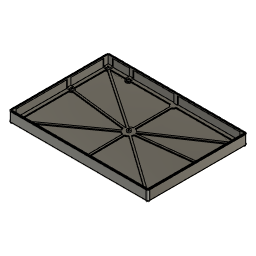
bottom (Autodesk Fusion 360 design; units mm, degrees)
Autodesk Fusion 360 part; units mm, degrees
note: some values were not read from the file. Set by a fixed rule: which sketch regions a step uses.
sketch "Szkic1" plane through (0, 0, 0) normal (0, 0, 1) x (1, 0, 0)
  line L0 (-4, -4) -> (301, -4)
  line L1 (301, -4) -> (301, 214)
  line L2 (301, 214) -> (-4, 214)
  line L3 (-4, 214) -> (-4, -4)
  circle A0 centre (5, 205) radius 1.6
  circle A1 centre (50, 205) radius 1.6
  circle A2 centre (292, 205) radius 1.6
  circle A3 centre (292, 5) radius 1.6
  circle A4 centre (148.5, 5) radius 1.6
  circle A5 centre (5, 5) radius 1.6
  circle A6 centre (147.5, 108) radius 1.6
  circle A7 centre (5, 125) radius 1.6
  circle A8 centre (292, 125) radius 1.6
  dimension "d1" = 4
  dimension "d2" = 4
  dimension "d3" = 214
  dimension "d4" = 301
  dimension "d5" = 3.2
  dimension "d6" = 3.2
  dimension "d7" = 3.2
  dimension "d8" = 3.2
  dimension "d9" = 3.2
  dimension "d10" = 3.2
  dimension "d11" = 3.2
  dimension "d12" = 3.2
  dimension "d13" = 3.2
  dimension "d14" = 205
  dimension "d15" = 5
  dimension "d16" = 50
  dimension "d17" = 292
  dimension "d18" = 5
  dimension "d19" = 5
  dimension "d20" = 148.5
  dimension "d22" = 292
  dimension "d24" = 125
  dimension "d25" = 108
  dimension "d26" = 147.5
  constraint horizontal L0
  constraint vertical L1
  constraint horizontal L2
  constraint vertical L3
  constraint horizontal A0.centre A1.centre
  constraint horizontal A1.centre A2.centre
  constraint horizontal A4.centre A5.centre
  constraint horizontal A3.centre A4.centre
  constraint horizontal A7.centre A8.centre
  constraint vertical A3.centre A8.centre
  constraint vertical A5.centre A7.centre
  measures "d1" horizontal distance of origin L0.start
  measures "d2" vertical distance of origin L0.start
  measures "d3" vertical distance of origin L2.end
  measures "d4" horizontal distance of origin L0.end
  measures "d5" diameter of A0
  measures "d6" diameter of A1
  measures "d7" diameter of A7
  measures "d8" diameter of A6
  measures "d9" diameter of A8
  measures "d10" diameter of A2
  measures "d11" diameter of A5
  measures "d12" diameter of A4
  measures "d13" diameter of A3
  measures "d14" vertical distance of origin A0.centre
  measures "d15" horizontal distance of origin A0.centre
  measures "d16" horizontal distance of origin A1.centre
  measures "d17" horizontal distance of origin A2.centre
  measures "d18" horizontal distance of origin A5.centre
  measures "d19" vertical distance of origin A5.centre
  measures "d20" horizontal distance of origin A4.centre
  measures "d22" horizontal distance of origin A8.centre
  measures "d24" vertical distance of origin A7.centre
  measures "d25" vertical distance of origin A6.centre
  measures "d26" horizontal distance of origin A6.centre
extrude "Wyciągnięcie proste1" add sketch "Szkic1" along normal blind 4
sketch "Szkic2" plane through (0, 0, 0) normal (0, 0, -1) x (1, 0, 0)
  circle A0 centre (292, -205) radius 1.6
  circle A1 centre (5, -205) radius 1.6
  circle A2 centre (50, -205) radius 1.6
  circle A3 centre (292, -5) radius 1.6
  circle A4 centre (148.5, -5) radius 1.6
  circle A5 centre (5, -5) radius 1.6
  circle A6 centre (147.5, -108) radius 1.6
  circle A7 centre (5, -125) radius 1.6
  circle A8 centre (292, -125) radius 1.6
  line L0 (-4, 4) -> (-4, -214)
  line L1 (-4, -214) -> (301, -214)
  line L2 (301, -214) -> (301, 4)
  line L3 (301, 4) -> (-4, 4)
  circle A9 centre (5, -5) radius 3
  circle A10 centre (148.5, -5) radius 3
  circle A11 centre (292, -5) radius 3
  circle A12 centre (292, -125) radius 3
  circle A13 centre (147.5, -108) radius 3
  circle A14 centre (5, -125) radius 3
  circle A15 centre (5, -205) radius 3
  circle A16 centre (50, -205) radius 3
  circle A17 centre (292, -205) radius 3
  dimension "d29" = 6
  dimension "d30" = 6
  dimension "d31" = 6
  dimension "d32" = 6
  dimension "d33" = 6
  dimension "d34" = 6
  dimension "d35" = 6
  dimension "d36" = 6
  dimension "d37" = 6
  constraint concentric A5 A9
  constraint concentric A4 A10
  constraint concentric A3 A11
  constraint concentric A8 A12
  constraint concentric A6 A13
  constraint concentric A7 A14
  constraint concentric A1 A15
  constraint concentric A2 A16
  constraint concentric A0 A17
  measures "d29" diameter of A9
  measures "d30" diameter of A10
  measures "d31" diameter of A11
  measures "d32" diameter of A12
  measures "d33" diameter of A13
  measures "d34" diameter of A14
  measures "d35" diameter of A15
  measures "d36" diameter of A16
  measures "d37" diameter of A17
extrude "Wyciągnięcie proste2" cut sketch "Szkic2" against normal blind 2 contours A9 | A10 | A11 | A12 | A13 | A14 | A15 | A16 | A17
sketch "Szkic3" plane through (0, 0, 4) normal (0, 0, 1) x (-1, 0, 0)
  circle A0 centre (-292, -205) radius 1.6
  circle A1 centre (-5, -205) radius 1.6
  circle A2 centre (-50, -205) radius 1.6
  circle A3 centre (-292, -5) radius 1.6
  circle A4 centre (-148.5, -5) radius 1.6
  circle A5 centre (-5, -5) radius 1.6
  circle A6 centre (-147.5, -108) radius 1.6
  circle A7 centre (-5, -125) radius 1.6
  circle A8 centre (-292, -125) radius 1.6
  line L0 (4, -214) -> (4, 4)
  line L1 (4, 4) -> (-301, 4)
  line L2 (-301, 4) -> (-301, -214)
  line L3 (-301, -214) -> (4, -214)
  circle A9 centre (-5, -205) radius 6
  circle A10 centre (-50, -205) radius 6
  circle A11 centre (-147.5, -108) radius 12
  circle A12 centre (-5, -125) radius 6
  circle A13 centre (-5, -5) radius 6
  circle A14 centre (-292, -205) radius 6
  circle A15 centre (-292, -125) radius 6
  circle A16 centre (-148.5, -5) radius 6
  circle A17 centre (-292, -5) radius 6
  line L4 (-5, -205) -> (-147.5, -108)
  line L5 (-147.5, -108) -> (-5, -125)
  line L6 (-5, -125) -> (-5, -205)
  line L7 (-5, -5) -> (-5, -125)
  line L8 (-5, -5) -> (-147.5, -108)
  line L9 (-147.5, -108) -> (-148.5, -5)
  line L10 (-148.5, -5) -> (-5, -5)
  line L11 (-148.5, -5) -> (-292, -5)
  line L12 (-292, -5) -> (-147.5, -108)
  line L13 (-147.5, -108) -> (-292, -125)
  line L14 (-292, -125) -> (-292, -5)
  line L15 (-292, -125) -> (-292, -205)
  line L16 (-292, -205) -> (-147.5, -108)
  line L17 (-5, -205) -> (-50, -205)
  line L18 (-50, -205) -> (-292, -205)
  circle A18 centre (-147.5, -205) radius 6
  line L19 (-147.5, -108) -> (-147.5, -205)
  line L20 (-10.8017, -203.4702) -> (-138.8443, -116.3113)
  line L21 (-145.5, -119.8322) -> (-145.5, -199.3431)
  line L22 (-149.5, -119.8322) -> (-149.5, -199.3431)
  line L23 (-286.1885, -203.5077) -> (-156.2093, -116.2552)
  line L24 (-288.4179, -200.1866) -> (-158.4387, -112.9341)
  line L25 (-159.0174, -111.3688) -> (-286.1482, -126.3253)
  line L26 (-286.6156, -122.3527) -> (-159.4848, -107.3962)
  line L27 (-158.2959, -102.7608) -> (-288.5545, -9.9121)
  line L28 (-286.2327, -6.6548) -> (-155.9741, -99.5036)
  line L29 (-149.6148, -96.1878) -> (-150.445, -10.676)
  line L30 (-146.4452, -10.6372) -> (-145.615, -96.149)
  line L31 (-139.0822, -99.4478) -> (-10.7562, -6.6929)
  line L32 (-8.413, -9.9347) -> (-136.739, -102.6896)
  line L33 (-10.3801, -122.344) -> (-135.5142, -107.4157)
  line L34 (-10.8539, -126.3158) -> (-135.9881, -111.3875)
  line L35 (-8.5509, -200.1635) -> (-136.5935, -113.0047)
  dimension "d40" = 12
  dimension "d41" = 12
  dimension "d42" = 24
  dimension "d43" = 12
  dimension "d44" = 12
  dimension "d45" = 12
  dimension "d46" = 12
  dimension "d47" = 12
  dimension "d48" = 12
  dimension "d49" = 12
  dimension "d50" = 2
  dimension "d51" = 2
  dimension "d52" = 2
  dimension "d53" = 2
  dimension "d54" = 2
  dimension "d55" = 2
  dimension "d56" = 2
  dimension "d57" = 2
  dimension "d58" = 2
  dimension "d59" = 2
  dimension "d60" = 2
  dimension "d61" = 2
  dimension "d62" = 2
  dimension "d63" = 2
  dimension "d64" = 2
  dimension "d65" = 2
  constraint concentric A1 A9
  constraint concentric A2 A10
  constraint concentric A6 A11
  constraint concentric A7 A12
  constraint concentric A5 A13
  constraint concentric A0 A14
  constraint concentric A8 A15
  constraint concentric A4 A16
  constraint concentric A3 A17
  constraint coincident A1.centre A9.centre
  constraint coincident A6.centre A11.centre
  constraint coincident A7.centre A12.centre
  constraint coincident A5.centre A13.centre
  constraint coincident A4.centre A16.centre
  constraint coincident A3.centre A17.centre
  constraint coincident A8.centre A15.centre
  constraint coincident A0.centre A14.centre
  constraint coincident A2.centre A10.centre
  constraint coincident L18 A18.centre
  constraint coincident A18.centre L19.end
  constraint coincident A9 L20.start
  constraint coincident A11 L20.end
  constraint parallel L4 L20
  constraint perpendicular L18 L19
  constraint coincident A11 L21.start
  constraint coincident A18 L21.end
  constraint parallel L19 L21
  constraint coincident A11 L22.start
  constraint coincident A18 L22.end
  constraint parallel L19 L22
  constraint coincident A14 L23.start
  constraint coincident A11 L23.end
  constraint parallel L16 L23
  constraint coincident A14 L24.start
  constraint coincident A11 L24.end
  constraint parallel L16 L24
  constraint coincident A11 L25.start
  constraint coincident A15 L25.end
  constraint parallel L13 L25
  constraint coincident A15 L26.start
  constraint parallel L25 L26
  constraint coincident A11 L26.end
  constraint coincident A11 L27.start
  constraint coincident A17 L27.end
  constraint parallel L12 L27
  constraint coincident A17 L28.start
  constraint coincident A11 L28.end
  constraint parallel L12 L28
  constraint coincident A11 L29.start
  constraint coincident A16 L29.end
  constraint parallel L9 L29
  constraint coincident A16 L30.start
  constraint coincident A11 L30.end
  constraint parallel L29 L30
  constraint coincident A11 L31.start
  constraint coincident A13 L31.end
  constraint parallel L8 L31
  constraint coincident A13 L32.start
  constraint coincident A11 L32.end
  constraint parallel L31 L32
  constraint coincident A12 L33.start
  constraint coincident A11 L33.end
  constraint parallel L5 L33
  constraint coincident A12 L34.start
  constraint coincident A11 L34.end
  constraint parallel L5 L34
  constraint coincident A9 L35.start
  constraint coincident A11 L35.end
  constraint parallel L4 L35
  measures "d40" diameter of A9
  measures "d41" diameter of A10
  measures "d42" diameter of A11
  measures "d43" diameter of A12
  measures "d44" diameter of A13
  measures "d45" diameter of A14
  measures "d46" diameter of A15
  measures "d47" diameter of A16
  measures "d48" diameter of A17
  measures "d49" diameter of A18
  measures "d50" distance of L4 L20
  measures "d51" distance of L4 L35
  measures "d52" distance of L19 L21
  measures "d53" distance of L19 L22
  measures "d54" distance of L16 L23
  measures "d55" distance of L16 L24
  measures "d56" distance of L13 L25
  measures "d57" distance of L13 L26
  measures "d58" distance of L12 L27
  measures "d59" distance of L12 L28
  measures "d60" distance of L9 L29
  measures "d61" distance of L9 L30
  measures "d62" distance of L8 L31
  measures "d63" distance of L8 L32
  measures "d64" distance of L5 L33
  measures "d65" distance of L5 L34
extrude "Wyciągnięcie proste3" cut sketch "Szkic3" against normal blind 2 contours A11 A14 L18 A18 L22 L23 | A11 A14 A15 L15 L24 L25 | A9 A10 A11 L17 L18 A18 L20 L21 | A11 A15 A17 L14 L26 L27 | A11 A16 A17 L11 L28 L29 | A9 A11 A12 L6 L34 L35 | A11 A12 A13 L7 L32 L33 | A11 A13 A16 L10 L30 L31
sketch "Szkic4" plane through (0, 0, 4) normal (0, 0, 1) x (-1, 0, 0)
  arc A0 (-135.5142, -107.4157) -> (-136.739, -102.6896) centre (-147.5, -108) ccw
  line L0 (-136.739, -102.6896) -> (-8.413, -9.9347)
  arc A1 (-8.413, -9.9347) -> (-5, -11) centre (-5, -5) ccw
  line L1 (-5, -11) -> (-5, -119)
  arc A2 (-5, -119) -> (-10.3801, -122.344) centre (-5, -125) ccw
  line L2 (-10.3801, -122.344) -> (-135.5142, -107.4157)
  arc A3 (-159.0174, -111.3688) -> (-158.4387, -112.9341) centre (-147.5, -108) ccw
  line L3 (-158.4387, -112.9341) -> (-288.4179, -200.1866)
  arc A4 (-288.4179, -200.1866) -> (-292, -199) centre (-292, -205) ccw
  line L4 (-292, -199) -> (-292, -131)
  arc A5 (-292, -131) -> (-286.1482, -126.3253) centre (-292, -125) ccw
  line L5 (-286.1482, -126.3253) -> (-159.0174, -111.3688)
  arc A6 (-158.2959, -102.7608) -> (-159.4848, -107.3962) centre (-147.5, -108) ccw
  line L6 (-159.4848, -107.3962) -> (-286.6156, -122.3527)
  arc A7 (-286.6156, -122.3527) -> (-292, -119) centre (-292, -125) ccw
  line L7 (-292, -119) -> (-292, -11)
  arc A8 (-292, -11) -> (-288.5545, -9.9121) centre (-292, -5) ccw
  line L8 (-288.5545, -9.9121) -> (-158.2959, -102.7608)
  arc A9 (-149.6148, -96.1878) -> (-155.9741, -99.5036) centre (-147.5, -108) ccw
  line L9 (-155.9741, -99.5036) -> (-286.2327, -6.6548)
  arc A10 (-286.2327, -6.6548) -> (-286, -5) centre (-292, -5) ccw
  line L10 (-286, -5) -> (-154.5, -5)
  arc A11 (-154.5, -5) -> (-150.445, -10.676) centre (-148.5, -5) ccw
  line L11 (-150.445, -10.676) -> (-149.6148, -96.1878)
  arc A12 (-136.5935, -113.0047) -> (-135.9881, -111.3875) centre (-147.5, -108) ccw
  line L12 (-135.9881, -111.3875) -> (-10.8539, -126.3158)
  arc A13 (-10.8539, -126.3158) -> (-5, -131) centre (-5, -125) ccw
  line L13 (-5, -131) -> (-5, -199)
  arc A14 (-5, -199) -> (-8.5509, -200.1635) centre (-5, -205) ccw
  line L14 (-8.5509, -200.1635) -> (-136.5935, -113.0047)
  line L15 (-153.5, -205) -> (-286, -205)
  arc A15 (-286, -205) -> (-286.1885, -203.5077) centre (-292, -205) ccw
  line L16 (-286.1885, -203.5077) -> (-156.2093, -116.2552)
  arc A16 (-156.2093, -116.2552) -> (-149.5, -119.8322) centre (-147.5, -108) ccw
  line L17 (-149.5, -119.8322) -> (-149.5, -199.3431)
  arc A17 (-149.5, -199.3431) -> (-153.5, -205) centre (-147.5, -205) ccw
  arc A18 (-145.5, -119.8322) -> (-138.8443, -116.3113) centre (-147.5, -108) ccw
  line L18 (-138.8443, -116.3113) -> (-10.8017, -203.4702)
  arc A19 (-10.8017, -203.4702) -> (-11, -205) centre (-5, -205) ccw
  line L19 (-11, -205) -> (-44, -205)
  arc A20 (-44, -205) -> (-56, -205) centre (-50, -205) ccw
  line L20 (-56, -205) -> (-141.5, -205)
  arc A21 (-141.5, -205) -> (-145.5, -199.3431) centre (-147.5, -205) ccw
  line L21 (-145.5, -199.3431) -> (-145.5, -119.8322)
  arc A22 (-139.0822, -99.4478) -> (-145.615, -96.149) centre (-147.5, -108) ccw
  line L22 (-145.615, -96.149) -> (-146.4452, -10.6372)
  arc A23 (-146.4452, -10.6372) -> (-142.5, -5) centre (-148.5, -5) ccw
  line L23 (-142.5, -5) -> (-11, -5)
  arc A24 (-11, -5) -> (-10.7562, -6.6929) centre (-5, -5) ccw
  line L24 (-10.7562, -6.6929) -> (-139.0822, -99.4478)
  circle A25 centre (-292, -205) radius 1.6
  circle A26 centre (-5, -205) radius 1.6
  circle A27 centre (-50, -205) radius 1.6
  circle A28 centre (-292, -5) radius 1.6
  circle A29 centre (-148.5, -5) radius 1.6
  circle A30 centre (-5, -5) radius 1.6
  circle A31 centre (-147.5, -108) radius 1.6
  circle A32 centre (-5, -125) radius 1.6
  circle A33 centre (-292, -125) radius 1.6
  line L25 (4, -214) -> (4, 4)
  line L26 (4, 4) -> (-301, 4)
  line L27 (-301, 4) -> (-301, -214)
  line L28 (-301, -214) -> (4, -214)
  line L29 (4, 4) -> (-301, 4)
  line L30 (-301, 4) -> (-301, -214)
  line L31 (-301, -214) -> (4, -214)
  line L32 (4, -214) -> (4, 4)
  circle A34 centre (-147.5, -108) radius 4
  line L33 (4, 4) -> (-301, 4)
  line L34 (-301, 4) -> (-301, -214)
  line L35 (-301, -214) -> (4, -214)
  line L36 (4, -214) -> (4, 4)
  line L37 (-288, -205) -> (-288, -212)
  line L38 (-292, -201) -> (-299, -201)
  arc A35 (-288, -205) -> (-292, -201) centre (-292, -205) ccw
  line L39 (-143.5, -210.5) -> (-143.5, -212)
  line L40 (-151.5, -210.5) -> (-151.5, -212)
  line L41 (-46, -205) -> (-46, -212)
  line L42 (-54, -205) -> (-54, -212)
  line L43 (-9, -205) -> (-9, -212)
  line L44 (-5, -201) -> (2, -201)
  line L45 (-5, -129) -> (2, -129)
  line L46 (-5, -121) -> (2, -121)
  line L47 (-5, -9) -> (2, -9)
  line L48 (-9, -5) -> (-9, 2)
  line L49 (-144.5, -5) -> (-144.5, 2)
  line L50 (-152.5, -5) -> (-152.5, 2)
  line L51 (-288, -5) -> (-288, 2)
  line L52 (-292, -9) -> (-299, -9)
  line L53 (-292, -121) -> (-299, -121)
  line L54 (-292, -129) -> (-299, -129)
  arc A36 (-292, -9) -> (-288, -5) centre (-292, -5) ccw
  line L55 (-9, 2) -> (-144.5, 2)
  line L56 (-152.5, 2) -> (-288, 2)
  arc A37 (-152.5, -5) -> (-144.5, -5) centre (-148.5, -5) ccw
  arc A38 (-9, -5) -> (-5, -9) centre (-5, -5) ccw
  line L57 (2, -201) -> (2, -129)
  line L58 (2, -121) -> (2, -9)
  arc A39 (-5, -121) -> (-5, -129) centre (-5, -125) ccw
  arc A40 (-5, -201) -> (-9, -205) centre (-5, -205) ccw
  line L59 (-46, -212) -> (-9, -212)
  arc A41 (-46, -205) -> (-54, -205) centre (-50, -205) ccw
  line L60 (-143.5, -210.5) -> (-151.5, -210.5)
  line L61 (-288, -212) -> (-151.5, -212)
  line L62 (-143.5, -212) -> (-54, -212)
  arc A42 (-292, -129) -> (-292, -121) centre (-292, -125) ccw
  line L63 (-299, -9) -> (-299, -121)
  line L64 (-299, -129) -> (-299, -201)
  dimension "d68" = 8
  dimension "d69" = 8
  dimension "d71" = 8
  dimension "d72" = 8
  dimension "d73" = 8
  dimension "d74" = 8
  dimension "d75" = 8
  dimension "d76" = 8
  dimension "d77" = 8
  dimension "d82" = 2
  dimension "d83" = 2
  dimension "d84" = 2
  dimension "d85" = 2
  dimension "d86" = 8
  dimension "d87" = 1.5
  dimension "d88" = 2
  constraint horizontal L29
  constraint vertical L30
  constraint horizontal L31
  constraint vertical L32
  constraint coincident L27.end L28.start
  constraint coincident L25.end L26.start
  constraint concentric A14 A40
  constraint concentric A20 A41
  constraint concentric A4 A35
  constraint concentric A0 A34
  constraint concentric A5 A42
  constraint concentric A8 A36
  constraint concentric A11 A37
  constraint concentric A1 A38
  constraint concentric A2 A39
  constraint horizontal L33
  constraint vertical L34
  constraint horizontal L35
  constraint vertical L36
  constraint horizontal L55
  constraint vertical L63
  constraint horizontal L61
  constraint vertical L57
  constraint perpendicular L37 L61
  constraint perpendicular L38 L63
  constraint tangent L37 A35
  constraint tangent L38 A35
  constraint coincident L39.end L61
  constraint perpendicular L39 L61
  constraint perpendicular L40 L61
  constraint coincident L41.end L61
  constraint tangent L41 A41
  constraint perpendicular L42 L61
  constraint tangent L42 A41
  constraint perpendicular L41 L61
  constraint tangent L43 A40
  constraint tangent L44 A40
  constraint tangent L45 A39
  constraint perpendicular L45 L57
  constraint coincident L46.end L57
  constraint tangent L46 A39
  constraint perpendicular L46 L57
  constraint tangent L47 A38
  constraint perpendicular L47 L57
  constraint tangent L48 A38
  constraint perpendicular L48 L55
  constraint tangent L49 A37
  constraint perpendicular L49 L55
  constraint coincident L50.end L55
  constraint tangent L50 A37
  constraint perpendicular L50 L55
  constraint tangent L51 A36
  constraint perpendicular L51 L55
  constraint perpendicular L52 L63
  constraint perpendicular L53 L63
  constraint coincident L54.end L63
  constraint perpendicular L54 L63
  constraint tangent L54 A42
  constraint tangent L53 A42
  constraint perpendicular L44 L57
  constraint perpendicular L43 L61
  constraint tangent L52 A36
  constraint collinear L55 L56
  constraint collinear L57 L58
  constraint collinear L59 L61
  constraint perpendicular L40 L60
  constraint collinear L61 L62
  constraint collinear L63 L64
  measures "d68" diameter of A40
  measures "d69" diameter of A41
  measures "d71" diameter of A35
  measures "d72" diameter of A34
  measures "d73" diameter of A42
  measures "d74" diameter of A36
  measures "d75" diameter of A37
  measures "d76" diameter of A38
  measures "d77" diameter of A39
  measures "d82" distance of L30 L63
  measures "d83" distance of L29 L55
  measures "d84" distance of L32 L58
  measures "d85" distance of L31 L59
  measures "d86" distance of L39 L40
  measures "d87" distance of L60 L62
  measures "d88" distance of L21 L39
extrude "Wyciągnięcie proste4" add sketch "Szkic4" along normal blind 3 contours L25 L26 L27 L28 L29 L30 L31 L32 L33 L34 L35 L36 | A34
sketch "Szkic5" plane through (0, 0, 7) normal (0, 0, 1) x (-1, 0, 0)
  circle A0 centre (-50, -205) radius 1.6
  line L0 (-299, -129) -> (-292, -129)
  arc A1 (-292, -129) -> (-292, -121) centre (-292, -125) ccw
  line L1 (-292, -121) -> (-299, -121)
  line L2 (-299, -121) -> (-299, -9)
  line L3 (-299, -9) -> (-292, -9)
  arc A2 (-292, -9) -> (-288, -5) centre (-292, -5) ccw
  line L4 (-288, -5) -> (-288, 2)
  line L5 (-288, 2) -> (-152.5, 2)
  line L6 (-152.5, 2) -> (-152.5, -5)
  arc A3 (-152.5, -5) -> (-144.5, -5) centre (-148.5, -5) ccw
  line L7 (-144.5, -5) -> (-144.5, 2)
  line L8 (-144.5, 2) -> (-9, 2)
  line L9 (-9, 2) -> (-9, -5)
  arc A4 (-9, -5) -> (-5, -9) centre (-5, -5) ccw
  line L10 (-5, -9) -> (2, -9)
  line L11 (2, -9) -> (2, -121)
  line L12 (2, -121) -> (-5, -121)
  arc A5 (-5, -121) -> (-5, -129) centre (-5, -125) ccw
  line L13 (-5, -129) -> (2, -129)
  line L14 (2, -129) -> (2, -201)
  line L15 (2, -201) -> (-5, -201)
  arc A6 (-5, -201) -> (-9, -205) centre (-5, -205) ccw
  line L16 (-9, -205) -> (-9, -212)
  line L17 (-9, -212) -> (-46, -212)
  line L18 (-46, -212) -> (-46, -205)
  arc A7 (-46, -205) -> (-54, -205) centre (-50, -205) ccw
  line L19 (-54, -205) -> (-54, -212)
  line L20 (-54, -212) -> (-143.5, -212)
  line L21 (-143.5, -212) -> (-143.5, -210.5)
  line L22 (-143.5, -210.5) -> (-151.5, -210.5)
  line L23 (-151.5, -210.5) -> (-151.5, -212)
  line L24 (-151.5, -212) -> (-288, -212)
  line L25 (-288, -212) -> (-288, -205)
  arc A8 (-288, -205) -> (-292, -201) centre (-292, -205) ccw
  line L26 (-292, -201) -> (-299, -201)
  line L27 (-299, -201) -> (-299, -129)
  circle A9 centre (-292, -205) radius 1.6
  circle A10 centre (-5, -5) radius 1.6
  circle A11 centre (-292, -125) radius 1.6
  circle A12 centre (-5, -125) radius 1.6
  circle A13 centre (-5, -205) radius 1.6
  circle A14 centre (-292, -5) radius 1.6
  circle A15 centre (-148.5, -5) radius 1.6
  line L28 (4, -214) -> (4, 4)
  line L29 (4, 4) -> (-301, 4)
  line L30 (-301, 4) -> (-301, -214)
  line L31 (-301, -214) -> (4, -214)
  line L32 (4, 4) -> (-301, 4)
  line L33 (-301, 4) -> (-301, -214)
  line L34 (-301, -214) -> (4, -214)
  line L35 (4, -214) -> (4, 4)
  line L36 (-9, 2) -> (-9, 0.5)
  line L37 (0.5, 0.5) -> (0.5, -9)
  line L38 (2, -9) -> (2, -121)
  line L39 (0.5, -121) -> (0.5, -129)
  line L40 (2, -129) -> (2, -201)
  line L41 (0.5, -201) -> (0.5, -210.5)
  line L42 (0.5, -210.5) -> (-9.123, -210.5)
  line L43 (-9, -212) -> (-46, -212)
  line L44 (-46, -210.5) -> (-54, -210.5)
  line L45 (-54, -212) -> (-143.5, -212)
  line L46 (-143.5, -210.5) -> (-151.5, -210.5)
  line L47 (-151.5, -212) -> (-288, -212)
  line L48 (-288, -210.5) -> (-297.5, -210.5)
  line L49 (-297.5, -210.5) -> (-297.5, -201)
  line L50 (-299, -201) -> (-299, -129)
  line L51 (-297.5, -129) -> (-297.5, -121)
  line L52 (-299, -121) -> (-299, -9)
  line L53 (-297.5, -9) -> (-297.5, 0.5)
  line L54 (-297.5, 0.5) -> (-288, 0.5)
  line L55 (-288, 2) -> (-152.5, 2)
  line L56 (-152.5, 0.5) -> (-144.5, 0.5)
  line L57 (-144.5, 2) -> (-9, 2)
  line L58 (0.5, 0.5) -> (-9, 0.5)
  dimension "d91" = 1.5
  dimension "d92" = 1.5
  dimension "d93" = 1.5
  dimension "d94" = 1.5
  dimension "d95" = 1.5
  dimension "d96" = 1.5
  dimension "d97" = 1.5
  dimension "d98" = 1.5
  dimension "d99" = 1.5
  dimension "d100" = 1.5
  dimension "d101" = 1.5
  dimension "d109" = 1.5
  constraint horizontal L32
  constraint vertical L33
  constraint horizontal L34
  constraint vertical L35
  constraint coincident L30.end L31.start
  constraint coincident L28.end L29.start
  constraint coincident L8.end L9.start
  constraint coincident L9 L36.end
  constraint perpendicular L8 L36
  constraint coincident L10 L37.end
  constraint perpendicular L10 L37
  constraint coincident L10.end L11.start
  constraint coincident L11.end L12.start
  constraint coincident L12 L39.start
  constraint coincident L13 L39.end
  constraint perpendicular L13 L39
  constraint coincident L13.end L14.start
  constraint coincident L14.end L15.start
  constraint coincident L15 L41.start
  constraint perpendicular L15 L41
  constraint perpendicular L41 L42
  constraint coincident L16.end L17.start
  constraint coincident L17.end L18.start
  constraint coincident L18 L44.start
  constraint coincident L19 L44.end
  constraint perpendicular L19 L44
  constraint coincident L19.end L20.start
  constraint coincident L20.end L21.start
  constraint coincident L21.end L22.start
  constraint coincident L22.end L23.start
  constraint coincident L23.end L24.start
  constraint coincident L24.end L25.start
  constraint coincident L25 L48.start
  constraint perpendicular L25 L48
  constraint coincident L26 L49.end
  constraint perpendicular L26 L49
  constraint coincident L26.end L27.start
  constraint coincident L0.start L27.end
  constraint coincident L0 L51.start
  constraint coincident L1 L51.end
  constraint perpendicular L1 L51
  constraint coincident L1.end L2.start
  constraint coincident L2.end L3.start
  constraint coincident L3 L53.start
  constraint perpendicular L3 L53
  constraint coincident L4 L54.end
  constraint perpendicular L4 L54
  constraint coincident L4.end L5.start
  constraint coincident L5.end L6.start
  constraint coincident L6 L56.start
  constraint coincident L7 L56.end
  constraint perpendicular L7 L56
  constraint coincident L7.end L8.start
  constraint perpendicular L9 L58
  measures "d91" distance of L42 L43
  measures "d92" distance of L40 L41
  measures "d93" distance of L43 L44
  measures "d94" distance of L49 L50
  measures "d95" distance of L47 L48
  measures "d96" distance of L50 L51
  measures "d97" distance of L52 L53
  measures "d98" distance of L54 L55
  measures "d99" distance of L56 L57
  measures "d100" distance of L57 L58
  measures "d101" distance of L37 L38
  measures "d109" distance of L39 L40
extrude "Wyciągnięcie proste5" add sketch "Szkic5" along normal blind 14.9 contours L28 L29 L30 L31 L32 L33 L34 L35
sketch "Szkic6" plane through (0, 0, 21.9) normal (0, 0, 1) x (-1, 0, 0)
  line L0 (0.5, 0.5) -> (0.5, -9)
  line L1 (0.5, -9) -> (2, -9)
  line L2 (2, -9) -> (2, -121)
  line L3 (2, -121) -> (0.5, -121)
  line L4 (0.5, -121) -> (0.5, -129)
  line L5 (0.5, -129) -> (2, -129)
  line L6 (2, -129) -> (2, -201)
  line L7 (2, -201) -> (0.5, -201)
  line L8 (0.5, -201) -> (0.5, -210.5)
  line L9 (0.5, -210.5) -> (-9, -210.5)
  line L10 (-9, -210.5) -> (-9, -212)
  line L11 (-9, -212) -> (-46, -212)
  line L12 (-46, -212) -> (-46, -210.5)
  line L13 (-46, -210.5) -> (-54, -210.5)
  line L14 (-54, -210.5) -> (-54, -212)
  line L15 (-54, -212) -> (-143.5, -212)
  line L16 (-143.5, -212) -> (-143.5, -210.5)
  line L17 (-143.5, -210.5) -> (-151.5, -210.5)
  line L18 (-151.5, -210.5) -> (-151.5, -212)
  line L19 (-151.5, -212) -> (-288, -212)
  line L20 (-288, -212) -> (-288, -210.5)
  line L21 (-288, -210.5) -> (-297.5, -210.5)
  line L22 (-297.5, -210.5) -> (-297.5, -201)
  line L23 (-297.5, -201) -> (-299, -201)
  line L24 (-299, -201) -> (-299, -129)
  line L25 (-299, -129) -> (-297.5, -129)
  line L26 (-297.5, -129) -> (-297.5, -121)
  line L27 (-297.5, -121) -> (-299, -121)
  line L28 (-299, -121) -> (-299, -9)
  line L29 (-299, -9) -> (-297.5, -9)
  line L30 (-297.5, -9) -> (-297.5, 0.5)
  line L31 (-297.5, 0.5) -> (-288, 0.5)
  line L32 (-288, 0.5) -> (-288, 2)
  line L33 (-288, 2) -> (-152.5, 2)
  line L34 (-152.5, 2) -> (-152.5, 0.5)
  line L35 (-152.5, 0.5) -> (-144.5, 0.5)
  line L36 (-144.5, 0.5) -> (-144.5, 2)
  line L37 (-144.5, 2) -> (-9, 2)
  line L38 (-9, 2) -> (-9, 0.5)
  line L39 (-9, 0.5) -> (0.5, 0.5)
  line L40 (4, -214) -> (4, 4)
  line L41 (4, 4) -> (-301, 4)
  line L42 (-301, 4) -> (-301, -214)
  line L43 (-301, -214) -> (4, -214)
  line L44 (4, 4) -> (-301, 4)
  line L45 (-301, 4) -> (-301, -214)
  line L46 (-301, -214) -> (4, -214)
  line L47 (4, -214) -> (4, 4)
  line L48 (-297.5, -210.5) -> (0.5, -210.5)
  line L49 (0.5, -210.5) -> (0.5, 0.5)
  line L50 (0.5, 0.5) -> (-297.5, 0.5)
  line L51 (-297.5, 0.5) -> (-297.5, -210.5)
  dimension "d104" = 3.5
  dimension "d105" = 3.5
  dimension "d107" = 3.5
  dimension "d108" = 3.5
  constraint horizontal L44
  constraint vertical L45
  constraint horizontal L46
  constraint vertical L47
  constraint coincident L42.end L43.start
  constraint coincident L40.end L41.start
  constraint horizontal L48
  constraint vertical L49
  constraint horizontal L50
  constraint vertical L51
  measures "d104" distance of L40.end L49
  measures "d105" distance of L44 L50
  measures "d107" distance of L46 L48
  measures "d108" distance of L45 L51
extrude "Wyciągnięcie proste6" add sketch "Szkic6" along normal blind 2 contours L1 L2 L3 L49 | L36 L37 L38 L50 | L5 L6 L7 L49 | L32 L33 L34 L50 | L10 L11 L12 L48 | L27 L28 L29 L51 | L14 L15 L16 L48 | L23 L24 L25 L51 | L18 L19 L20 L48 | L40 L41 L42 L43 L44 L45 L46 L47
sketch "Szkic7" plane through (0, 0, 23.9) normal (0, 0, 1) x (-1, 0, 0)
  line L0 (-297.5, -210.5) -> (-297.5, 0.5)
  line L1 (-297.5, 0.5) -> (0.5, 0.5)
  line L2 (0.5, 0.5) -> (0.5, -210.5)
  line L3 (0.5, -210.5) -> (-297.5, -210.5)
  line L4 (4, -214) -> (4, 4)
  line L5 (4, 4) -> (-301, 4)
  line L6 (-301, 4) -> (-301, -214)
  line L7 (-301, -214) -> (4, -214)
  line L8 (0.5, -210.5) -> (-297.5, -210.5)
  line L9 (-297.5, -210.5) -> (-297.5, 0.5)
  line L10 (-297.5, 0.5) -> (0.5, 0.5)
  line L11 (0.5, 0.5) -> (0.5, -210.5)
  line L12 (0.5, -212.1) -> (-297.5, -212.1)
  line L13 (-299.1, -210.5) -> (-299.1, 0.5)
  line L14 (-297.5, 2.1) -> (0.5, 2.1)
  line L15 (2.1, 0.5) -> (2.1, -210.5)
  arc A0 (2.1, 0.5) -> (0.5, 2.1) centre (0.5, 0.5) ccw
  arc A1 (0.5, -212.1) -> (2.1, -210.5) centre (0.5, -210.5) ccw
  arc A2 (-299.1, -210.5) -> (-297.5, -212.1) centre (-297.5, -210.5) ccw
  arc A3 (-297.5, 2.1) -> (-299.1, 0.5) centre (-297.5, 0.5) ccw
  dimension "d112" = 1.6
  dimension "d113" = 1.6
  dimension "d114" = 1.6
  dimension "d115" = 1.6
  dimension "d142" = 3.2
  dimension "d143" = 3.2
  dimension "d144" = 3.2
  dimension "d145" = 3.2
  constraint horizontal L8
  constraint vertical L9
  constraint horizontal L10
  constraint vertical L11
  constraint coincident L0.end L1.start
  constraint coincident L2.end L3.start
  constraint horizontal L12
  constraint vertical L13
  constraint horizontal L14
  constraint vertical L15
  constraint coincident L1.end L2.start
  constraint coincident L0.start L3.end
  measures "d112" distance of L11 L15
  measures "d113" distance of L10 L14
  measures "d114" distance of L8 L12
  measures "d115" distance of L9 L13
  measures "d142" diameter of A0
  measures "d143" diameter of A1
  measures "d144" diameter of A2
  measures "d145" diameter of A3
extrude "Wyciągnięcie proste7" add sketch "Szkic7" along normal blind 0.8 contours L12 L13 L14 L15 A0 A1 A2 A3
sketch "Szkic8" plane through (0, 0, 0) normal (0, 0, -1) x (1, 0, 0)
  circle A0 centre (292, -205) radius 3
  circle A1 centre (148.5, -5) radius 3
  circle A2 centre (5, -5) radius 3
  circle A3 centre (292, -5) radius 3
  circle A4 centre (50, -205) radius 3
  circle A5 centre (292, -125) radius 3
  circle A6 centre (5, -125) radius 3
  circle A7 centre (147.5, -108) radius 3
  circle A8 centre (5, -205) radius 3
  line L0 (-4, 4) -> (-4, -214)
  line L1 (-4, -214) -> (301, -214)
  line L2 (301, -214) -> (301, 4)
  line L3 (301, 4) -> (-4, 4)
  line L4 (15.9, -2.4) -> (36.1, -2.4)
  line L5 (36.1, -2.4) -> (36.1, -7.6)
  line L6 (36.1, -7.6) -> (15.9, -7.6)
  line L7 (15.9, -7.6) -> (15.9, -2.4)
  line L8 (137.4, -96.4) -> (157.6, -96.4)
  line L9 (137.4, -101.6) -> (137.4, -96.4)
  line L10 (157.6, -96.4) -> (157.6, -101.6)
  line L11 (157.6, -101.6) -> (137.4, -101.6)
  line L12 (15.9, -202.4) -> (36.1, -202.4)
  line L13 (15.9, -207.6) -> (15.9, -202.4)
  line L14 (36.1, -202.4) -> (36.1, -207.6)
  line L15 (36.1, -207.6) -> (15.9, -207.6)
  line L16 (260.9, -207.6) -> (260.9, -202.4)
  line L17 (260.9, -202.4) -> (281.1, -202.4)
  line L18 (281.1, -202.4) -> (281.1, -207.6)
  line L19 (281.1, -207.6) -> (260.9, -207.6)
  line L20 (260.9, -7.6) -> (260.9, -2.4)
  line L21 (260.9, -2.4) -> (281.1, -2.4)
  line L22 (281.1, -2.4) -> (281.1, -7.6)
  line L23 (281.1, -7.6) -> (260.9, -7.6)
  dimension "d118" = 20.2
  dimension "d119" = 5.2
  dimension "d120" = 20.2
  dimension "d121" = 5.2
  dimension "d122" = 20.2
  dimension "d123" = 5.2
  dimension "d124" = 20.2
  dimension "d125" = 5.2
  dimension "d126" = 20.2
  dimension "d127" = 5.2
  dimension "d128" = 6.4
  dimension "d129" = 19.9
  dimension "d130" = 6.4
  dimension "d131" = 6.4
  dimension "d132" = 6.4
  dimension "d133" = 19.9
  dimension "d134" = 19.9
  dimension "d135" = 19.9
  dimension "d136" = 10.1
  dimension "d137" = 6.4
  constraint horizontal L4
  constraint vertical L5
  constraint horizontal L6
  constraint vertical L7
  constraint horizontal L8
  constraint vertical L10
  constraint horizontal L11
  constraint vertical L9
  constraint horizontal L12
  constraint vertical L14
  constraint horizontal L15
  constraint vertical L13
  constraint horizontal L17
  constraint vertical L18
  constraint horizontal L19
  constraint vertical L16
  constraint horizontal L21
  constraint vertical L22
  constraint horizontal L23
  constraint vertical L20
  measures "d118" distance of L5.end L6.end
  measures "d119" distance of L4.end L5.end
  measures "d120" distance of L10.end L9.start
  measures "d121" distance of L10.end L8.end
  measures "d122" distance of L14.end L13.start
  measures "d123" distance of L14.end L12.end
  measures "d124" distance of L16.start L18.end
  measures "d125" distance of L18.end L17.end
  measures "d126" distance of L20.start L22.end
  measures "d127" distance of L22.end L21.end
  measures "d128" distance of L1 L15
  measures "d129" distance of L0 L13
  measures "d130" distance of L3 L4
  measures "d131" distance of L3 L21
  measures "d132" distance of L1 L19
  measures "d133" distance of L0 L7
  measures "d134" distance of L2 L22
  measures "d135" distance of L2 L18
  measures "d136" distance of A7.centre L10
  measures "d137" distance of A7.centre L11
extrude "Wyciągnięcie proste8" cut sketch "Szkic8" against normal blind 0.3 contours L4 L5 L6 L7 | L8 L9 L10 L11 | L12 L13 L14 L15 | L16 L17 L18 L19 | L20 L21 L22 L23
fillet "Zaokrąglenie1" radius 4 8 edges at (148.5, 214, 0) (-4, 214, 11.95) (-4, 105, 0) (148.5, -4, 0) (-4, -4, 11.95) (301, 214, 11.95) (301, 105, 0) (301, -4, 11.95)
